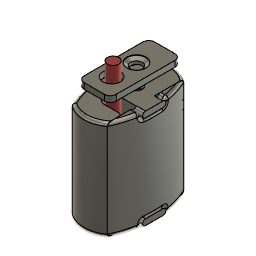
toolhead_scewmount v1 (Autodesk Fusion 360 design; units mm, degrees)
part number: MainBody
Autodesk Fusion 360 part; units mm, degrees
sketch "Sketch1" plane through (0, 0, 0) normal (0, 1, 0) x (1, 0, 0)
  line L0 (0, 0) -> (11, 0)
  line L1 (11, 0) -> (11, 24.2)
  line L2 (9, 24.2) -> (2, 24.2)
  line L3 (0, 22.2) -> (0, 0)
  line L4 (5.5, 0) -> (5.5, 6.5)
  circle A0 centre (5.5, 6.5) radius 2
  line L5 (11, 24.2) -> (0, 24.2)
  line L6 (0, 24.2) -> (0, 14.2)
  line L7 (2, 12.2) -> (9, 12.2)
  line L8 (11, 14.2) -> (11, 22.2)
  arc A1 (2, 24.2) -> (0, 22.2) centre (2, 22.2) ccw
  arc A2 (0, 14.2) -> (2, 12.2) centre (2, 14.2) ccw
  arc A3 (11, 22.2) -> (9, 24.2) centre (9, 22.2) ccw
  arc A4 (9, 12.2) -> (11, 14.2) centre (9, 14.2) ccw
  line L9 (11, 12.2) -> (0, 12.2)
  point P0 (0, 24.2)
  point P1 (11, 12.2)
  dimension "d1" = 11
  dimension "d2" = 24.2
  dimension "d3" = 6.5
  dimension "d4" = 4
  dimension "d5" = 12
  dimension "d10" = 2
  dimension "d11" = 2
  dimension "d12" = 2
  constraint horizontal L0
  constraint vertical L1
  constraint horizontal L2
  constraint vertical L3
  constraint coincident L0.start L3.end
  constraint midpoint L0 L4.start
  constraint perpendicular L0 L4
  constraint coincident L4.end A0.centre
  constraint horizontal L5
  constraint vertical L6
  constraint horizontal L7
  constraint vertical L8
  constraint coincident P0 L2
  constraint coincident P0 L3
  constraint tangent L2 A1
  constraint tangent L3 A1
  constraint tangent L6 A2
  constraint tangent L7 A2
  constraint equal A1 A2
  constraint coincident L1.end L2
  constraint coincident L1.end L8
  constraint tangent L2 A3
  constraint tangent L8 A3
  constraint coincident P1 L7
  constraint coincident P1 L8
  constraint tangent L7 A4
  constraint tangent L8 A4
  constraint coincident P1 L9.start
  constraint coincident L3 L9.end
  constraint perpendicular L3 L9
  measures "d1" distance of L0.start L0.end
  measures "d2" distance of L0.start P0
  measures "d3" distance of L4.start L4.end
  measures "d4" diameter of A0
  measures "d5" distance of L1.end P1
  measures "d10" radius of A1
  measures "d11" radius of A3
  measures "d12" radius of A4
extrude "Extrude1" add sketch "Sketch1" against normal blind 4 contours L0 L1 L3 L7 L9 | L3 A2 L9 | L1 L2 L3 L5 L6 L7 L8 A1 A2 A3 A4 L9 | L1 A4 L9 | L5 L6 A1 | L1 L5 A3 | A0 makes body 1
extrude "Extrude2" add sketch "Sketch1" along normal blind 5 contours L0 L1 L3 L7 L9 bodies 1
extrude "Extrude3" add sketch "Sketch1" along normal blind 18 contours L1 L2 L3 L5 L6 L7 L8 A1 A2 A3 A4 L9 bodies 1
extrude "Extrude4" add sketch "Sketch1" along normal blind 40 contours A0 bodies 1
sketch "Sketch1 (2)" plane through (0, -4, 0) normal (0, -1, 0) x (1, 0, 0) in component "MainBody"
  line L0 (11, -24.2) -> (11, 0)
  line L1 (11, 0) -> (0, 0)
  line L2 (0, 0) -> (0, -24.2)
  line L3 (0, -24.2) -> (11, -24.2)
  line L4 (0, -12.1) -> (-4, -12.1) construction
  line L5 (0, 0) -> (-1, 0) construction
  line L6 (-1, 0) -> (-1, 1) construction
  line L7 (-1, 1) -> (0, 1) construction
  line L8 (0, 1) -> (0, 0) construction
  line L9 (0, -24.2) -> (-1, -24.2) construction
  line L10 (-1, -24.2) -> (-1, -25.2) construction
  line L11 (-1, -25.2) -> (0, -25.2) construction
  line L12 (0, -25.2) -> (0, -24.2) construction
  line L13 (11, -24.2) -> (11, -25.2)
  line L14 (5.5, -24.2) -> (5.5, -27.2) construction
  line L15 (11, 0) -> (11, 1)
  line L16 (5.5, 0) -> (5.5, 3) construction
  arc A0 (11, 1) -> (-1, 1) centre (5, -6.9375) ccw
  arc A1 (-1, -25.2) -> (11, -25.2) centre (5, -17.2625) ccw
  arc A2 (-1, 1) -> (-1, -25.2) centre (26.1017, -12.1) ccw
  dimension "d17" = 4
  dimension "d93" = 1
  dimension "d94" = 1
  dimension "d95" = 1
  dimension "d96" = 1
  dimension "d97" = 1
  dimension "d98" = 3
  dimension "d99" = 1
  dimension "d100" = 3
  constraint midpoint L2 L4.start
  constraint perpendicular L2 L4
  constraint horizontal L5
  constraint vertical L6
  constraint horizontal L7
  constraint vertical L8
  constraint coincident L1.end L2.start
  constraint horizontal L9
  constraint vertical L10
  constraint horizontal L11
  constraint vertical L12
  constraint coincident L2.end L3.start
  constraint coincident L0.start L3.end
  constraint perpendicular L3 L13
  constraint midpoint L3 L14.start
  constraint perpendicular L3 L14
  constraint coincident L0.end L1.start
  constraint perpendicular L1 L15
  constraint midpoint L1 L16.start
  constraint perpendicular L1 L16
  constraint coincident L16.end A0
  constraint coincident L14.end A1
  constraint coincident L4.end A2
  measures "d17" distance of L4.start L4.end
  measures "d93" distance of L1.end L5.end
  measures "d94" distance of L1.end L7.end
  measures "d95" distance of L2.end L9.end
  measures "d96" distance of L2.end L11.end
  measures "d97" distance of L0.start L13.end
  measures "d98" distance of L14.start L14.end
  measures "d99" distance of L0.end L15.end
  measures "d100" distance of L16.start L16.end
extrude "Extrude1'" add sketch "Sketch1 (2)" along normal blind 2 separate body makes body 2 in component "MainBody"
extrude "Extrude2'" add sketch "Sketch1 (2)" against normal blind 26 contours L1 L2 L3 L13 L15 A0 A1 A2 bodies 2 in component "MainBody"
sketch "Sketch2" plane through (0, 0, 0) normal (1, 0, 0) x (0, 0, -1) in component "MainBody"
  line L0 (24.2, 22) -> (0, 22)
  line L1 (24.2, -4) -> (24.2, 22)
  line L2 (0, 22) -> (0, -4)
  line L3 (0, -4) -> (24.2, -4)
  line L4 (0, 22) -> (11.8, 22)
  line L5 (11.8, 22) -> (11.8, 5.2)
  line L6 (11.8, 5.2) -> (0, 5.2)
  line L7 (0, 5.2) -> (0, 22)
  line L8 (0, 22) -> (4, 22)
  line L9 (11.8, 5.2) -> (9, 5.2)
  line L10 (9, 5.2) -> (4, 5.2)
  line L11 (4, 5.2) -> (4, 22)
  line L12 (4, 22) -> (9, 22)
  line L13 (9, 22) -> (9, 5.2)
  dimension "d101" = 11.8
  dimension "d102" = 16.8
  dimension "d103" = 4
  dimension "d104" = 2.8
  constraint horizontal L4
  constraint vertical L5
  constraint horizontal L6
  constraint vertical L7
  constraint coincident L0.end L2.start
  constraint perpendicular L7 L8
  constraint perpendicular L5 L9
  constraint horizontal L10
  constraint vertical L11
  constraint horizontal L12
  constraint vertical L13
  measures "d101" distance of L0.end L4.end
  measures "d102" distance of L0.end L6.end
  measures "d103" distance of L0.end L8.end
  measures "d104" distance of L5.end L9.end
extrude "Extrude3'" add sketch "Sketch2" along normal blind 11 separate body contours L0 L4 L5 L6 L9 L13 | L0 L2 L4 L6 L7 L8 L11 makes body 3 at (3.6667, 16.4, -9) makes body 4 at (3.6667, 10.8, -4) in component "MainBody"
sketch "Sketch3" plane through (0, 22, 0) normal (0, 1, 0) x (-1, 0, 0) in component "MainBody"
  line L0 (0, 0) -> (0, -24.2)
  line L1 (-11, 0) -> (-7.8688, 0)
  line L2 (-5, 0) -> (-5, -6.5)
  circle A0 centre (-5, -6.5) radius 2.5
  line L3 (0, -24.2) -> (-11, -24.2)
  line L4 (-11, 0) -> (0, 0)
  line L5 (-11, 1) -> (-11, 0)
  line L6 (-11, -24.2) -> (-11, -25.2)
  arc A1 (-11, -25.2) -> (1, -25.2) centre (-5, -17.2625) ccw
  arc A2 (1, -25.2) -> (1, 1) centre (-26.1017, -12.1) ccw
  arc A3 (1, 1) -> (-11, 1) centre (-5, -6.9375) ccw
  line L7 (-11, -24.2) -> (0, -24.2)
  line L8 (0, -24.2) -> (0, 0)
  line L9 (0, 0) -> (-11, 0)
  line L10 (-11, 0) -> (-11, -24.2)
  dimension "d35" = 6.5
  dimension "d36" = 5
  constraint horizontal L1
  constraint coincident L1.start L4.start
  constraint coincident L2.end A0.centre
  constraint horizontal L7
  constraint vertical L8
  constraint horizontal L9
  constraint vertical L10
  constraint coincident L0.start L4.end
  constraint coincident L3.end L6.start
  measures "d35" distance of L2.start L2.end
  measures "d36" diameter of A0
extrude "Extrude4'" add sketch "Sketch3" along normal blind 6 bodies 3 4 2 in component "MainBody"
sketch "Sketch4" plane through (0, 28, 0) normal (0, 1, 0) x (-1, 0, 0) in component "MainBody"
  line L0 (-5, -6) -> (-5, -15)
  circle A0 centre (-5, -15) radius 2
  arc A1 (-11, -25.2) -> (1, -25.2) centre (-5, -17.2625) ccw
  arc A2 (1, -25.2) -> (1, 1) centre (-26.1017, -12.1) ccw
  arc A3 (1, 1) -> (-11, 1) centre (-5, -6.9375) ccw
  line L1 (-11, 1) -> (-11, -25.2)
  circle A4 centre (-5, -6.5) radius 2.5
  dimension "d37" = 9
  dimension "d38" = 4
  constraint vertical L0
  constraint coincident L0.end A0.centre
  measures "d37" distance of L0.start L0.end
  measures "d38" diameter of A0
extrude "Extrude5" cut sketch "Sketch4" against normal blind 6 contours A0 bodies 3 in component "MainBody"
sketch "Sketch5" plane through (11, 0, 0) normal (1, 0, 0) x (0, 0, -1) in component "MainBody"
  line L0 (15, 28) -> (15, 26)
  line L1 (15, 26) -> (17.8, 26)
  line L2 (17.8, 26) -> (12.2, 26)
  line L3 (12.2, 26) -> (12.2, 23)
  line L4 (12.2, 23) -> (17.8, 23)
  line L5 (17.8, 23) -> (17.8, 26)
  line L6 (0, 5.2) -> (4, 5.2)
  line L7 (11.8, 5.2) -> (11.8, 22)
  line L8 (9, 22) -> (9, 5.2)
  line L9 (0, -4) -> (0, 5.2)
  line L10 (4, 22) -> (9, 22)
  line L11 (4, 5.2) -> (4, 22)
  line L12 (25.2, -6) -> (25.2, 28)
  line L13 (25.2, 28) -> (-1, 28)
  line L14 (-1, 28) -> (-1, -6)
  line L15 (-1, -6) -> (25.2, -6)
  line L16 (24.2, 22) -> (24.2, -4)
  line L17 (24.2, -4) -> (0, -4)
  line L18 (9, 5.2) -> (11.8, 5.2)
  line L19 (11.8, 22) -> (24.2, 22)
  dimension "d42" = 2
  dimension "d43" = 2.8
  dimension "d44" = 5.6
  dimension "d45" = 3
  constraint perpendicular L0 L1
  constraint horizontal L2
  constraint vertical L3
  constraint horizontal L4
  constraint vertical L5
  measures "d42" distance of L0.start L0.end
  measures "d43" distance of L0.end L1.end
  measures "d44" distance of L1.end L2.end
  measures "d45" distance of L1.end L4.end
extrude "Extrude6" cut sketch "Sketch5" against normal blind 10 contours L1 L2 L3 L4 L5 bodies 3 in component "MainBody"
sketch "Sketch1 (3)" plane through (0, 28, 0) normal (0, 1, 0) x (-1, 0, 0) in component "lid"
  line L0 (-10.9479, -11.7913) -> (-13.9467, -11.7064)
  arc A0 (-11, 1) -> (-11, -25.2) centre (16.6195, -12.1) ccw
  arc A1 (-11, -25.2) -> (1, -25.2) centre (-5, -17.2625) ccw
  arc A2 (1, -25.2) -> (1, 1) centre (-26.1017, -12.1) ccw
  arc A3 (1, 1) -> (-11, 1) centre (-5, -6.9375) ccw
  line L1 (-11, 1) -> (-11, -25.2)
  circle A4 centre (-5, -15) radius 2
  circle A5 centre (-5, -6.5) radius 2.5
  dimension "d48" = 3
  constraint coincident L0.end A0
  constraint coincident A0.start A3.end
  constraint coincident A0.end A1.start
  measures "d48" distance of L0.start L0.end
extrude "Extrude1''" add sketch "Sketch1 (3)" against normal blind 34 separate body contours L0 A0 L1 | L0 A0 L1 makes body 5 in component "lid"
sketch "Sketch6" plane through (0, 0, -24.2) normal (0, 0, 1) x (1, 0, 0) in component "MainBody"
  line L0 (11, 22) -> (5, 22)
  line L1 (5, 22) -> (5, 19)
  line L2 (5, 19) -> (11, 19)
  line L3 (11, 19) -> (11, 22)
  line L4 (11, -4) -> (11, 22)
  line L5 (0, 22) -> (0, -4)
  line L6 (0, -4) -> (11, -4)
  line L7 (11, 22) -> (0, 22)
  dimension "d52" = 3
  constraint horizontal L0
  constraint vertical L1
  constraint horizontal L2
  constraint vertical L3
  constraint coincident L0.start L3.end
  measures "d52" distance of L2.end L0.start
extrude "Extrude7" cut sketch "Sketch6" against normal blind 4 contours L0 L1 L2 L3 L4 L7 bodies 3 in component "MainBody"
fillet "Fillet1" radius 2 2 edges at (1, 24.5, -12.2) (1, 24.5, -17.8) on bodies 3 in component "MainBody"
fillet "Fillet2" radius 1 2 edges at (11, 24.5, -12.2) (11, 24.5, -17.8) on bodies 3 in component "MainBody"
fillet "Fillet3" radius 2 2 edges at (0, 13.6, -9) (0, 13.6, -4) on bodies 3 in component "MainBody"
fillet "Fillet8" radius 1 1 edges at (11, 13.6, -11.8) on bodies 3 in component "MainBody"
fillet "Fillet9" radius 1 2 edges at (5, 20.5, -27.2126) (5, 20.5, -24.2) on bodies 3 in component "MainBody"
fillet "Fillet10" radius 1 7 edges at (0, 22, -18) (5, 22, -11.8) (10.7071, 22, -11.5071) (2, 22, -24.2) (4.7071, 22, -24.4929) (5, 22, -25.6783) (4.6664, 22, -26.9021) on bodies 3 in component "MainBody"
fillet "Fillet11" radius 1 3 edges at (4.7071, 19, -24.4929) (5, 19, -25.6783) (4.6664, 19, -26.9021) on bodies 3 in component "MainBody"
sketch "Sketch11" plane through (11, 0, 0) normal (1, 0, 0) x (0, 0, -1) in component "MainBody"
  line L0 (12.5321, 22) -> (25.2, 22)
  line L1 (25.2, 22) -> (25.2, 28)
  line L2 (25.2, 28) -> (-1, 28)
  line L3 (-1, 28) -> (-1, -6)
  line L4 (-1, -6) -> (25.2, -6)
  line L5 (25.2, -6) -> (25.2, 19)
  line L6 (25.2, 19) -> (24.2, 19)
  line L7 (24.2, 19) -> (24.2, -4)
  line L8 (24.2, -4) -> (0, -4)
  line L9 (0, -4) -> (0, 5.2)
  line L10 (0, 5.2) -> (4, 5.2)
  line L11 (4, 5.2) -> (4, 22)
  line L12 (4, 22) -> (9, 22)
  line L13 (9, 22) -> (9, 5.2)
  line L14 (9, 5.2) -> (10.8, 5.2)
  line L15 (10.8, 5.2) -> (10.8, 21)
  spline S0 degree 3 poles (12.5321, 22) (12.2772, 22) (11.9847, 21.9104) (11.4152, 21.6039) (11.0771, 21.2771) (10.8, 21) knots 0.505532 0.505532 0.505532 0.505532 0.581995 0.581995 0.699558 0.699558 0.699558 0.699558
  line L16 (18.8, 23) -> (11.2, 23)
  line L17 (11.2, 23) -> (11.2, 26)
  line L18 (11.2, 26) -> (18.8, 26)
  line L19 (18.8, 26) -> (18.8, 23)
  line L20 (12.1, 28) -> (12.1, 27)
  line L21 (12.1, 27) -> (15.1, 27)
  line L22 (12.1, 27) -> (9.1, 27)
  circle A0 centre (15.1, 27) radius 1
  circle A1 centre (9.1, 27) radius 1
  line L23 (9.1, 26) -> (15, 26)
  line L24 (12.1, -6) -> (12.1, -5)
  line L25 (12.1, -5) -> (12.19, -5)
  line L26 (12.1, -5) -> (15.1, -5)
  circle A2 centre (15.1, -5) radius 1
  line L27 (12.1, -5) -> (9.1, -5)
  circle A3 centre (9.1, -5) radius 1
  dimension "d131" = 1
  dimension "d132" = 3
  dimension "d133" = 3
  dimension "d134" = 1
  dimension "d136" = 3
  dimension "d157" = 3
  constraint midpoint L2 L20.start
  constraint perpendicular L2 L20
  constraint perpendicular L20 L21
  constraint perpendicular L20 L22
  constraint coincident L21.end A0.centre
  constraint tangent L2 A0
  constraint coincident L22.end A1.centre
  constraint tangent L2 A1
  constraint coincident A1 L23.start
  constraint midpoint L18 L23.end
  constraint tangent A0 L23
  constraint midpoint L4 L24.start
  constraint perpendicular L4 L24
  constraint perpendicular L24 L25
  constraint perpendicular L24 L26
  constraint coincident L26.end A2.centre
  constraint tangent L4 A2
  constraint perpendicular L24 L27
  constraint coincident L27.end A3.centre
  constraint tangent L4 A3
  measures "d131" distance of L20.start L20.end
  measures "d132" distance of L20.end L21.end
  measures "d133" distance of L20.end L22.end
  measures "d134" distance of L24.start L24.end
  measures "d136" distance of L24.end L26.end
  measures "d157" distance of L24.end L27.end
extrude "Extrude12" add sketch "Sketch11" along normal blind 3 contours L2 L20 L21 A0 | A0 | L2 L20 L22 A1 | L18 L21 L22 A0 A1 L23 | A1 | L4 L24 L27 A3 | A3 | L4 L24 L25 L26 A2 | L8 L25 L26 A2 L27 A3 | A2 bodies 3 in component "MainBody"
sketch "Sketch3 (2)" plane through (11, 0, 0) normal (-1, 0, 0) x (0, 0, 1) in component "lid"
  line L0 (1, 28) -> (-25.2, 28)
  line L1 (-25.2, 28) -> (-25.2, -6)
  line L2 (-25.2, -6) -> (1, -6)
  line L3 (1, -6) -> (1, 28)
  line L4 (-12.1, 28) -> (-12.1, 26.9)
  line L5 (-12.1, 26.9) -> (-9, 26.9)
  line L6 (-12.1, 26.9) -> (-15.2, 26.9)
  circle A0 centre (-15.2, 26.9) radius 1.1
  circle A1 centre (-9, 26.9) radius 1.1
  line L7 (-9, 25.8) -> (-15.2, 25.8)
  line L8 (-16.3, 26.9) -> (-7.9, 26.9)
  line L9 (-7.9, 26.9) -> (-7.9, 28)
  line L10 (-7.9, 28) -> (-16.3, 28)
  line L11 (-16.3, 28) -> (-16.3, 26.9)
  line L12 (-12.1, -6) -> (-12.1, -5)
  line L13 (-12.1, -5) -> (-9, -5)
  line L14 (-12.1, -5) -> (-15.2, -5)
  circle A2 centre (-15.2, -5) radius 1
  circle A3 centre (-9, -5) radius 1
  line L15 (-15.2, -4) -> (-9, -4)
  line L16 (-8, -5) -> (-8, -6)
  line L17 (-16.2, -5) -> (-16.2, -6)
  dimension "d119" = 1.1
  dimension "d139" = 3.1
  dimension "d140" = 3.1
  dimension "d141" = 8.4
  dimension "d142" = 1
  dimension "d143" = 3.1
  dimension "d144" = 3.1
  constraint midpoint L0 L4.start
  constraint perpendicular L0 L4
  constraint perpendicular L4 L5
  constraint perpendicular L4 L6
  constraint coincident L6.end A0.centre
  constraint tangent L0 A0
  constraint coincident L5.end A1.centre
  constraint tangent L0 A1
  constraint coincident A1 L7.start
  constraint coincident A0 L7.end
  constraint tangent A0 L7
  constraint parallel L5 L7
  constraint horizontal L8
  constraint vertical L9
  constraint horizontal L10
  constraint vertical L11
  constraint coincident A0 L8.start
  constraint midpoint L2 L12.start
  constraint perpendicular L2 L12
  constraint perpendicular L12 L13
  constraint perpendicular L12 L14
  constraint coincident L14.end A2.centre
  constraint tangent L2 A2
  constraint coincident L13.end A3.centre
  constraint tangent L2 A3
  constraint coincident A2 L15.start
  constraint coincident A3 L15.end
  constraint tangent A3 L15
  constraint parallel L14 L15
  constraint coincident A3 L16.start
  constraint coincident L2 L16.end
  constraint tangent A3 L16
  constraint perpendicular L2 L16
  constraint coincident A2 L17.start
  constraint coincident L2 L17.end
  constraint tangent A2 L17
  constraint perpendicular L2 L17
  measures "d119" distance of L4.start L4.end
  measures "d139" distance of L4.end L5.end
  measures "d140" distance of L4.end L6.end
  measures "d141" distance of L8.start L8.end
  measures "d142" distance of L12.start L12.end
  measures "d143" distance of L12.end L13.end
  measures "d144" distance of L12.end L14.end
extrude "Extrude3''" cut sketch "Sketch3 (2)" against normal blind 4 contours L0 A1 L9 L10 | L0 L4 L5 A1 L8 L10 | L5 A1 L8 | L5 A1 L8 | L2 A3 L16 | L0 L4 L6 A0 L8 L10 | L5 L6 A0 A1 L7 L8 | L2 L12 L13 A3 | A3 | L0 A0 L10 L11 | L6 A0 L8 | L6 A0 L8 | L2 L12 L14 A2 | L13 L14 A2 A3 L15 | L2 A2 L17 | A2 bodies 5 in component "lid"
fillet "Fillet2'" radius 1 10 edges at (13.673, -5.5, -8) (13.7113, -4.292, -8.2938) (13.9492, -4, -12.1) (13.7113, -4.292, -15.9062) (13.673, -5.5, -16.2) (13.6593, 27.45, -16.3) (13.7024, 26.1212, -15.9768) (13.9492, 25.8, -12.1) (13.7024, 26.1212, -8.2232) (13.6593, 27.45, -7.9) on bodies 5 in component "lid"
sketch "Sketch13" plane through (11, 0, 0) normal (1, 0, 0) x (0, 0, -1) in component "MainBody"
  line L0 (-1, -6) -> (9.1, -6)
  line L1 (9.1, -4) -> (0, -4)
  line L2 (25.2, 22) -> (25.2, 28)
  line L3 (4, 22) -> (9, 22)
  line L4 (9, 22) -> (9, 28)
  line L5 (9, 28) -> (4, 28)
  line L6 (4, 28) -> (4, 22)
  arc A0 (9.1, 28) -> (9.1, 26) centre (9.1, 27) ccw
  line L7 (9.1, 28) -> (-1, 28)
  line L8 (-1, 28) -> (-1, -6)
  arc A1 (9.1, -4) -> (9.1, -6) centre (9.1, -5) ccw
  line L9 (0, -4) -> (0, 5.2)
  line L10 (0, 5.2) -> (4, 5.2)
  line L11 (4, 5.2) -> (4, 22)
  line L12 (4, 22) -> (9, 22)
  line L13 (9, 22) -> (9, 5.2)
  line L14 (9, 5.2) -> (10.8, 5.2)
  line L15 (10.8, 5.2) -> (10.8, 21)
  spline S0 degree 3 poles (12.5321, 22) (12.2772, 22) (11.9847, 21.9104) (11.4152, 21.6039) (11.0771, 21.2771) (10.8, 21) knots 0.505532 0.505532 0.505532 0.505532 0.581995 0.581995 0.699558 0.699558 0.699558 0.699558
  line L16 (12.5321, 22) -> (25.2, 22)
  line L17 (25.2, 28) -> (15.1, 28)
  arc A2 (15.1, 26) -> (15.1, 28) centre (15.1, 27) ccw
  line L18 (15.1, 26) -> (18.8, 26)
  line L19 (18.8, 26) -> (18.8, 23)
  line L20 (18.8, 23) -> (11.2, 23)
  line L21 (11.2, 23) -> (11.2, 26)
  line L22 (11.2, 26) -> (9.1, 26)
  dimension "d150" = 5
  constraint horizontal L3
  constraint vertical L4
  constraint horizontal L5
  constraint vertical L6
  constraint coincident L3.start L6.end
  measures "d150" distance of L3.end L3.start
extrude "Extrude14" cut sketch "Sketch13" against normal blind 6 contours L3 L4 L5 L6 A0 L7 L12 | L4 A0 bodies 3 in component "MainBody"
fillet "Fillet13" radius 1 6 edges at (3.5, 22, -4) (0.5858, 22, -4.5858) (0, 22, -6.5) (0.5858, 22, -8.4142) (3.5, 22, -9) (2.5, 22, -6.5) on bodies 3 in component "MainBody"
fillet "Fillet14" radius 1 2 edges at (11, 16.6, -4) (11, 15.6025, -9) on bodies 3 in component "MainBody"
fillet "Fillet15" radius 1 6 edges at (-4, -6, -12.1) (5, -6, 3.0126) (5, -6, -27.2126) (5, 28, -27.2126) (-4, 28, -12.1) (5, 28, 3.0126) on bodies 3 in component "MainBody"
fillet "Fillet3'" radius 1 12 edges at (12.4937, 28, -2.7797) (13.2552, 28, -7.5419) (11.7442, 28, -7.9) (11.7442, 28, -16.3) (13.2552, 28, -16.6581) (12.4937, 28, -21.4203) (11.753, -6, -8) (13.2717, -6, -7.6432) (12.5097, -6, -2.8297) (12.5097, -6, -21.3703) (13.2717, -6, -16.5568) (11.753, -6, -16.2) on bodies 5 in component "lid"
fillet "Fillet16" radius 1 10 edges at (11, 5.2, -1.5) (10.7071, 5.2, -3.7071) (6, 5.2, -4) (0.5858, 5.2, -4.5858) (0.5858, 5.2, -8.4142) (6, 5.2, -9) (10.7071, 5.2, -9.2929) (11, 5.2, -10.4) (10.7071, 5.2, -11.5071) (5, 5.2, -11.8) on bodies 3 in component "MainBody"
ref_plane "WorkPlane1" through (3.9545, 33, -12.1) normal (0, 1, 0) x (-1, 0, 0) in component "cover"
sketch "Sketch1 (4)" plane through (3.9545, 33, -12.1) normal (0, 1, 0) x (1, 0, 0) in component "cover"
  line L0 (0, 0) -> (1.05, 0)
  line L1 (1.05, 0) -> (1.05, 2.9)
  circle A0 centre (1.05, 2.9) radius 2
  line L2 (0, 0) -> (-3.95, 0)
  line L3 (-3.95, 0) -> (-3.95, 12.1)
  line L4 (-3.95, 12.1) -> (7.05, 12.1)
  line L5 (7.05, 12.1) -> (7.05, -12.05)
  line L6 (7.05, -12.05) -> (-3.95, -12.05)
  line L7 (-3.95, -12.05) -> (-3.95, 12.1)
  line L8 (1.05, 2.9) -> (1.05, -5.6)
  circle A1 centre (1.05, -5.6) radius 3
  dimension "d165" = 1.05
  dimension "d166" = 2.9
  dimension "d167" = 4
  dimension "d168" = 3.95
  dimension "d169" = 12.1
  dimension "d170" = 11
  dimension "d171" = 24.15
  dimension "d172" = 8.5
  dimension "d173" = 6
  constraint coincident L0.start L2.start
  constraint horizontal L0
  constraint perpendicular L0 L1
  constraint coincident L1.end A0.centre
  constraint parallel L0 L2
  constraint perpendicular L2 L3
  constraint horizontal L4
  constraint vertical L5
  constraint horizontal L6
  constraint vertical L7
  constraint parallel L1 L8
  constraint coincident L8.end A1.centre
  measures "d165" distance of L0.start L0.end
  measures "d166" distance of L0.end L1.end
  measures "d167" diameter of A0
  measures "d168" distance of L0.start L2.end
  measures "d169" distance of L2.end L3.end
  measures "d170" distance of L3.end L4.end
  measures "d171" distance of L3.end L6.end
  measures "d172" distance of L1.end L8.end
  measures "d173" diameter of A1
extrude "Extrude1'''" add sketch "Sketch1 (4)" along normal blind 2 separate body makes body 6 in component "cover"
hole "Hole1" at (5.0045, 35, -15) direction (0, -1, 0) diameter 6.5 depth 0.2 tip angle 118 bodies 6 in component "cover"
fillet "Fillet1'" radius 2 4 edges at (0.0045, 34, -0.05) (11.0045, 34, -0.05) (0.0045, 34, -24.2) (11.0045, 34, -24.2) on bodies 6 in component "cover"
component "MainBody" placed x (1, 0, 0) y (0, 1, 0) z (0, 0, 1) at (0, 0, 0)
component "cover" placed x (1, 0, 0) y (0, 1, 0) z (0, 0, 1) at (0, 0, 0)
component "lid" placed x (1, 0, 0) y (0, 1, 0) z (0, 0, 1) at (0, 0, 0) in component "MainBody"
equation "d8 = 9 mm - 4 mm"
equation "d13 = 20 mm - 2 mm"
equation "d44 = ( 2.8 * 2 ) * 1 mm"
